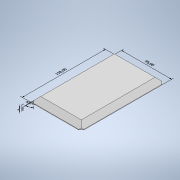
# Autodesk Inventor part: Деталь1
Saved by Autodesk Inventor 2021.2 (Build 252289000, 289)
## iProperties
Created: 2024-03-01
Part Number: Деталь1
Material: Типовые
Document SubType Name: Modeling
Designer: student
Density: 1 g/cm^3
Appearance: По умолчанию
Author: student
Autodesk Inventor part; units mm, degrees
ref_plane "YZ Plane" through (0, 0, 0) normal (1, 0, 0) x (0, 1, 0)
ref_plane "XZ Plane" through (0, 0, 0) normal (0, 1, 0) x (-1, 0, 0)
ref_plane "XY Plane" through (0, 0, 0) normal (0, 0, 1) x (1, 0, 0)
sketch "Эскиз1" plane through (0, 0, 0) normal (0, 1, 0) x (-1, 0, 0)
  line L0 (-47.5, 79) -> (47.5, 79)
  line L1 (47.5, 79) -> (47.5, -79)
  line L2 (47.5, -79) -> (-47.5, -79)
  line L3 (-47.5, -79) -> (-47.5, 79)
  line L4 (-47.5, 79) -> (47.5, -79) construction
  line L5 (47.5, 79) -> (-47.5, -79) construction
  point P0 (0, 0)
  dimension "d0" = 95
  dimension "d1" = 158
  constraints: 12 end point, 2 midpoint, 2 parallel, 1 horizontal, 1 perpendicular
  measures "d0" distance of L1.end L2.end
  measures "d1" distance of L0.end L1.end
extrude "Выдавливание1" add sketch "Эскиз1" along normal blind 10
chamfer "Фаска1" distance 5 angle 45 1 edges at (47.5, 5, 79) measured on face at (47.5, 6.6667, 26.3333)
chamfer "Фаска2" distance 5 angle 45 1 edges at (47.5, 5, -79) measured on face at (15.8333, 3.3333, -79)
chamfer "Фаска3" distance 5 angle 45 1 edges at (-47.5, 5, -79) measured on face at (12.5, 3.3333, -79)
chamfer "Фаска4" distance 5 angle 45 1 edges at (-47.5, 5, 79) measured on face at (-17.5, 3.3333, 79)
chamfer "Фаска5" distance 9 angle 45 1 edges at (-47.5, 10, 0) measured on face at (15.8333, 10, 24.6667)
chamfer "Фаска6" distance 9 angle 45 1 edges at (2, 10, -79) measured on face at (-9.8333, 10, -24.6667)
chamfer "Фаска7" distance 9 angle 45 1 edges at (47.5, 10, 2) measured on face at (-9.8333, 10, 27.6667)
chamfer "Фаска8" distance 9 angle 45 1 edges at (0, 10, 79) measured on face at (12.8333, 10, -20.3333)
